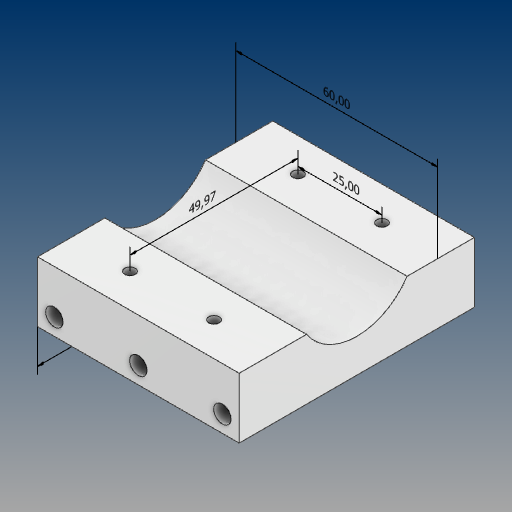
# Autodesk Inventor part: 18_Kep_han_A
Saved by Autodesk Inventor 2021 (Build 250183000, 183)
## iProperties
Created: 2024-04-05
Part Number: 18_Kep_han_A
Material: ABS Plastic
Document SubType Name: Modeling
Designer: Admin
Density: 1.06 g/cm^3
Appearance: Smooth - White
Author: Admin
Autodesk Inventor part; units mm, degrees
ref_plane "YZ Plane" through (0, 0, 0) normal (1, 0, 0) x (0, 1, 0)
ref_plane "XZ Plane" through (0, 0, 0) normal (0, 1, 0) x (-1, 0, 0)
ref_plane "XY Plane" through (0, 0, 0) normal (0, 0, 1) x (1, 0, 0)
sketch "Sketch1" plane through (0, 0, 0) normal (0, 1, 0) x (-1, 0, 0)
  line L0 (-30, 35) -> (30, 35)
  line L1 (30, 35) -> (30, -35)
  line L2 (30, -35) -> (-30, -35)
  line L3 (-30, -35) -> (-30, 35)
  line L4 (-30, 35) -> (30, -35) construction
  line L5 (30, 35) -> (-30, -35) construction
  point P0 (0, 0)
  dimension "d0" = 60
  dimension "d1" = 70
  constraints: 12 end point, 2 midpoint, 2 parallel, 1 horizontal, 1 perpendicular
  measures "d0" distance of L1.end L2.end
  measures "d1" distance of L0.end L1.end
extrude "Extrusion1" add sketch "Sketch1" along normal blind 18
sketch "Sketch2" plane through (30, 0, -35) normal (0, 0, -1) x (-1, 0, 0)
  line L0 (0, 0) -> (60, 0) projected
  line L1 (60, 0) -> (60, 18) projected
  line L2 (0, 18) -> (60, 18) projected
  line L3 (0, 0) -> (0, 18) projected
  line L4 (0, 5) -> (60, 5) construction
  line L5 (30, 0) -> (30, 18) construction
  line L6 (0, 18) -> (60, 18) projected
  point P0 (5, 5)
  point P1 (30, 5)
  point P2 (55, 5)
  dimension "d4" = 5
  dimension "d6" = 5
  constraints: 5 point on line, 4 end point, 2 midpoint, 1 horizontal, 1 symmetric about line
  measures "d4" distance between parallel lines of L0 L4
  measures "d6" distance from line of L1 point (55, 5)
hole "Hole1" at (25, 5, -35) at (0, 5, -35) at (-25, 5, -35) direction (0, 0, 1) diameter 5.2 end through all
sketch "Sketch3" plane through (30, 0, 35) normal (1, 0, 0) x (0, 0, -1)
  line L0 (0, 2.4) -> (70, 2.4) projected
  line L1 (0, 2.4) -> (0, 7.6) projected
  line L2 (70, 7.6) -> (70, 2.4) projected
  line L3 (0, 7.6) -> (70, 7.6) projected
  line L4 (0, 0) -> (70, 0) projected
  line L5 (70, 0) -> (70, 18) projected
  line L6 (0, 18) -> (70, 18) projected
  line L7 (0, 0) -> (0, 18) projected
  circle A0 centre (35, 28) radius 18
  point P0 (35, 0)
  point P1 (35, 0)
  point P2 (49.9666, 18)
  point P3 (20.0334, 18)
  dimension "d14" = 36
  dimension "d15" = 10
  constraints: 1 centre point, 1 midpoint, 1 vertical alignment
  measures "d14" diameter of A0
  measures "d15" distance from line of L6 A0.centre
extrude "Extrusion2" cut sketch "Sketch3" against normal through all contours L6 A0 picked at (30.9706, 16.8877)
sketch "Sketch4" plane through (0, 18, 0) normal (0, 1, 0) x (1, 0, 0)
  line L0 (-22.4, -35) -> (-27.6, -35) projected
  line L1 (-27.6, 35) -> (-22.4, 35) projected
  line L2 (2.6, -35) -> (-2.6, -35) projected
  line L3 (-2.6, 35) -> (2.6, 35) projected
  line L4 (27.6, -35) -> (22.4, -35) projected
  line L5 (22.4, 35) -> (27.6, 35) projected
  line L6 (-30, -35) -> (30, -35) projected
  line L7 (-12.5, -35) -> (-12.5, 35) construction
  line L8 (2.6, 35) -> (22.4, 35)
  line L9 (2.6, -35) -> (2.6, 35) projected
  line L10 (-22.4, 35) -> (-2.6, 35)
  line L11 (-22.4, -35) -> (-22.4, 35) projected
  line L12 (12.5, 35) -> (12.5, -35) construction
  line L13 (-30, -14.9666) -> (-30, -35) projected
  line L14 (-30, 35) -> (-30, 14.9666) projected
  line L15 (-30, 24.9833) -> (10, 24.9833) construction
  line L16 (-30, -24.9833) -> (30, -24.9833) construction
  line L17 (30, -35) -> (30, -14.9666) projected
  point P0 (0, 0)
  point P1 (-12.5, -24.9833)
  point P2 (12.5, -24.9833)
  point P3 (12.5, 24.9833)
  point P4 (-12.5, 24.9833)
  constraints: 12 end point, 8 point on line, 5 midpoint, 2 perpendicular, 2 vertical, 1 horizontal, 3 other
hole "Hole2" at (-12.5, 18, 24.9833) at (12.5, 18, 24.9833) at (12.5, 18, -24.9833) at (-12.5, 18, -24.9833) direction (0, -1, 0) diameter 3.2 end through all
body "Solid1"
